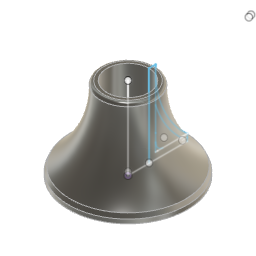
_32mm Magnet Hat.40945085-6c69-4d11-b43d-e7daac8e9fd8_LV0 (Autodesk Fusion 360 design; units mm, degrees)
Autodesk Fusion 360 part; units mm, degrees
sketch "Sketch1" plane through (0, 0, 0) normal (1, 0, 0) x (0, 1, 0)
  line L0 (6.4, 0) -> (6.4, 25)
  line L1 (0, 25) -> (0, 0)
  line L2 (6.4, 0.1899) -> (6.4, 25)
  line L3 (0, 0) -> (18, 0)
  line L4 (0, 1) -> (0, 0)
  line L5 (6.4, 25) -> (7.4, 25)
  line L6 (18, 0) -> (18, 1)
  line L7 (18, 1) -> (16.5, 1) construction
  line L8 (7.4, 25) -> (8.4, 25)
  line L9 (18, 1) -> (18, 2)
  arc A0 (8.4, 25) -> (18, 2) centre (37.363, 23.5854) ccw
  line L10 (8.4, 25) -> (8.4, 7)
  line L11 (18, 2) -> (9, 2)
  line L12 (18, 2) -> (16, 2)
  arc A1 (8.4, 14.3286) -> (16, 2) centre (36.7237, 23.282) ccw
  line L13 (8.4, 7) -> (8.4, 2)
  line L14 (8.4, 2) -> (9, 2)
  arc A2 (8.4, 4.5) -> (10.5136, 2) centre (10.9353, 4.5) ccw
  dimension "d1" = 6.4
  dimension "d2" = 25
  dimension "d10" = 1
  dimension "d11" = 1
  dimension "d14" = 1
  dimension "d15" = 1
  dimension "d16" = 2
  constraint vertical L0
  constraint vertical L1
  constraint coincident L1.end L3.start
  constraint vertical L2
  constraint horizontal L3
  constraint vertical L4
  constraint perpendicular L2 L5
  constraint perpendicular L3 L6
  constraint horizontal L7
  constraint perpendicular L1 L8
  constraint perpendicular L7 L9
  constraint perpendicular L8 L10
  constraint perpendicular L9 L11
  constraint perpendicular L9 L12
  constraint tangent A0 A1
  constraint coincident L10 A1.start
  constraint parallel L10 L13
  constraint perpendicular L10 L14
  constraint tangent L13 A2
  constraint coincident L11 A2.end
  constraint midpoint L13 A2.start
  measures "d1" distance of L1.end L0.start
  measures "d2" distance of L1.end L1.start
  measures "d10" distance of L0.end L5.end
  measures "d11" distance of L3.end L6.end
  measures "d14" distance of L5.end L8.end
  measures "d15" distance of L6.end L9.end
  measures "d16" distance of L9.end L12.end
revolve "Revolve3" add sketch "Sketch1" angle 360 about axis through (0, 0, 25) along (0, 0, -1) contours L0 L2 L3 L5 L6 L8 L9 A0 L10 L11 L12 L13 L14 | A0 L10 L11 L12 A1 | L11 L13 L14 A2
chamfer "Chamfer4" distance 0.75 angle 45 1 edges at (-16.7819, 6.5091, 2)
chamfer "Chamfer5" distance 0.5 angle 45 1 edges at (-5.9669, 2.3143, 0)
fillet "Fillet1" radius 1 1 edges at (-7.8315, 3.0376, 25)
